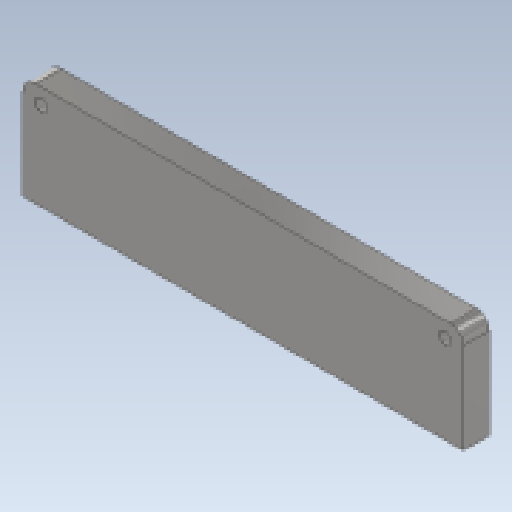
# Autodesk Inventor part: Support_driver
Saved by Autodesk Inventor 2025.2 (Build 292293000, 293)
## iProperties
Created: 2025-05-12
Part Number: Support_driver
Material: Stainless Steel
Document SubType Name: Modeling
Designer: Sergio Quintero
Density: 8 g/cm^3
Appearance: Semi-Polished
Author: Sergio Quintero
Autodesk Inventor part; units mm, degrees
ref_plane "YZ Plane" through (0, 0, 0) normal (1, 0, 0) x (0, 1, 0)
ref_plane "XZ Plane" through (0, 0, 0) normal (0, 1, 0) x (-1, 0, 0)
ref_plane "XY Plane" through (0, 0, 0) normal (0, 0, 1) x (1, 0, 0)
sketch "Sketch1" plane through (0, 0, 0) normal (0, 0, 1) x (1, 0, 0)
  line L0 (85, -20) -> (-85, -20)
  line L1 (-85, -20) -> (-85, 20)
  line L2 (-85, 20) -> (85, 20)
  line L3 (85, 20) -> (85, -20)
  line L4 (85, -20) -> (-85, 20) construction
  line L5 (-85, -20) -> (85, 20) construction
  point P0 (0, 0)
  dimension "d0" = 170
  dimension "d1" = 40
  constraints: 12 end point, 2 midpoint, 2 parallel, 1 horizontal, 1 perpendicular
  measures "d0" distance of L1.end L2.end
  measures "d1" distance of L0.end L1.end
extrude "Extrusion1" add sketch "Sketch1" along normal blind 10
sketch "Sketch2" plane through (0, 0, 10) normal (0, 0, 1) x (1, 0, 0)
  line L0 (85, 20) -> (-85, 20) construction
  line L1 (0, 20) -> (0, -20) construction
  line L2 (-85, -20) -> (85, -20) construction
  line L3 (-85, 20) -> (-85, -20) projected
  line L4 (85, -20) -> (85, 20) projected
  point P0 (0, 0)
  point P1 (-78, 14)
  point P2 (78, 14)
  dimension "d4" = 7
  dimension "d5" = 6
  constraints: 2 end point, 2 midpoint, 1 symmetric about line
  measures "d4" distance from line of L3 point (-78, 14)
  measures "d5" distance from line of point (-78, 14) L0
hole "Hole1" at (-78, 14, 10) at (78, 14, 10) direction (0, 0, -1) diameter 4.917 end through all thread size "M6x1" class "6H" standard "ISO Metric profile"
sketch "Sketch3" plane through (-85, -20, 0) normal (0, -1, 0) x (1, 0, 0)
  line L0 (0, 0) -> (0, 10) projected
  line L1 (0, 10) -> (170, 10) projected
  line L2 (85, 0) -> (85, 10) construction
  point P0 (7, 5)
  point P1 (0, 5)
  point P2 (163, 5)
  dimension "d24" = 5
  dimension "d25" = 7
  constraints: 2 end point, 2 midpoint, 1 symmetric about line
  measures "d24" distance from line of L1 point (7, 5)
  measures "d25" distance of point (0, 5) point (7, 5)
hole "Hole2" at (-78, -20, 5) at (78, -20, 5) direction (0, 1, 0) diameter 4.917 depth 15 tip angle 118 thread size "M6x1" class "6H" standard "ISO Metric profile"
fillet "Fillet1" radius 5 2 edges at (-85, 20, 5) (85, 20, 5)
body "Solid1"
